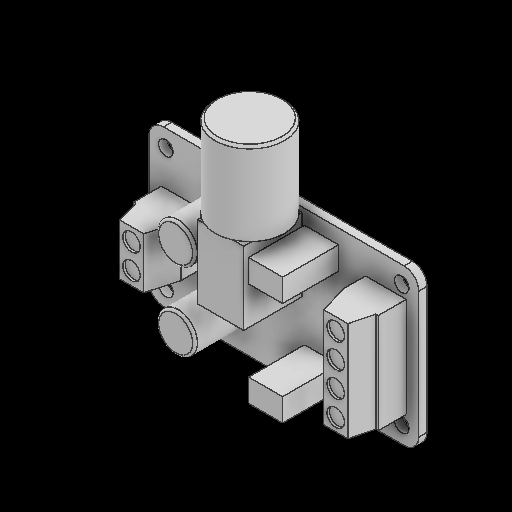
# Autodesk Inventor part: LQ-AMP10W
Saved by Autodesk Inventor 2025.2 (Build 292293000, 293)
## iProperties
Created: 2026-01-28
Part Number: LQ-AMP10W
Material: Generic
Document SubType Name: Modeling
Designer: valer
Density: 1 g/cm^3
Appearance: Default
Author: valer
Autodesk Inventor part; units mm, degrees
ref_plane "YZ Plane" through (0, 0, 0) normal (1, 0, 0) x (0, 1, 0)
ref_plane "XZ Plane" through (0, 0, 0) normal (0, 1, 0) x (-1, 0, 0)
ref_plane "XY Plane" through (0, 0, 0) normal (0, 0, 1) x (1, 0, 0)
sketch "Board" plane through (0, 0, 0) normal (0, 0, 1) x (1, 0, 0)
  line L0 (-27.75, 16) -> (27.75, 16)
  line L1 (27.75, 16) -> (27.75, -16)
  line L2 (27.75, -16) -> (-27.75, -16)
  line L3 (-27.75, -16) -> (-27.75, 16)
  line L4 (-27.75, 16) -> (27.75, -16) construction
  line L5 (27.75, 16) -> (-27.75, -16) construction
  line L6 (-24.25, -12.5) -> (24.25, -12.5) construction
  line L7 (24.25, -12.5) -> (24.25, 12.5) construction
  line L8 (24.25, 12.5) -> (-24.25, 12.5) construction
  line L9 (-24.25, 12.5) -> (-24.25, -12.5) construction
  line L10 (-24.25, -12.5) -> (24.25, 12.5) construction
  line L11 (24.25, -12.5) -> (-24.25, 12.5) construction
  circle A0 centre (24.25, 12.5) radius 1.5
  circle A1 centre (-24.25, 12.5) radius 1.5
  circle A2 centre (24.25, -12.5) radius 1.5
  circle A3 centre (-24.25, -12.5) radius 1.5
  line L12 (-25.75, -14) -> (-22.75, -14) construction
  line L13 (-22.75, -14) -> (-22.75, -11) construction
  line L14 (-22.75, -11) -> (-25.75, -11) construction
  line L15 (-25.75, -11) -> (-25.75, -14) construction
  line L16 (-25.75, -14) -> (-22.75, -11) construction
  line L17 (-22.75, -14) -> (-25.75, -11) construction
  point P0 (0, 0)
  dimension "d0" = 55.5
  dimension "d1" = 32
  dimension "d2" = 3
  dimension "d3" = 2
  dimension "d5" = 2
  dimension "d6" = 48.5
  constraints: 36 end point, 6 midpoint, 6 parallel, 4 centre point, 4 coincident, 3 equal radius, 3 horizontal, 3 perpendicular, 2 tangent
  measures "d0" distance of L0.start L0.end
  measures "d1" distance of L0.end L1.end
  measures "d2" diameter of A0
  measures "d3" distance between parallel lines of L2 L12
  measures "d5" distance between parallel lines of L3 L15
  measures "d6" distance of L7.end L8.end
extrude "BoardFeature" add sketch "Board" along normal blind 1.7
fillet "BoardFilletsFeature" radius 3 4 edges at (-27.75, 16, 0.85) (27.75, 16, 0.85) (-27.75, -16, 0.85) (27.75, -16, 0.85)
sketch "PotentiometerHousing" plane through (0, 0, 1.7) normal (0, 0, 1) x (1, 0, 0)
  line L0 (-5.75, 15) -> (3.75, 15)
  line L1 (3.75, 15) -> (3.75, 0)
  line L2 (3.75, 0) -> (-5.75, 0)
  line L3 (-5.75, 0) -> (-5.75, 15)
  line L4 (24.75, 16) -> (-24.75, 16) projected
  line L5 (-27.75, 13) -> (-27.75, -13) projected
  point P0 (0, 0)
  dimension "d10" = 1
  dimension "d11" = 22
  dimension "d12" = 15
  dimension "d13" = 9.5
  constraints: 8 end point, 2 parallel, 1 horizontal, 1 perpendicular
  measures "d10" distance between parallel lines of L4 L0
  measures "d11" distance between parallel lines of L5 L3
  measures "d12" distance of L0.end L1.end
  measures "d13" distance of L1.end L2.end
extrude "PotentiometerHousingFeature" add sketch "PotentiometerHousing" along normal blind 12
sketch "IJ63" plane through (0, 0, 1.7) normal (0, 0, 1) x (1, 0, 0)
  line L0 (4.25, 13) -> (11.25, 13)
  line L1 (11.25, 13) -> (11.25, 8.3)
  line L2 (11.25, 8.3) -> (4.25, 8.3)
  line L3 (4.25, 8.3) -> (4.25, 13)
  line L4 (3.75, 15) -> (-5.75, 15) projected
  line L5 (3.75, 0) -> (3.75, 15) projected
  line L6 (-38.85, 0) -> (38.85, 0) construction
  line L7 (4.25, -13) -> (11.25, -13)
  line L8 (11.25, -13) -> (11.25, -8.3)
  line L9 (11.25, -8.3) -> (4.25, -8.3)
  line L10 (4.25, -8.3) -> (4.25, -13)
  point P0 (0, 0)
  dimension "d16" = 2
  dimension "d17" = 4.7
  dimension "d18" = 7
  dimension "d19" = 0.5
  constraints: 16 end point, 4 symmetric about line, 2 parallel, 1 horizontal, 1 perpendicular
  measures "d16" distance between parallel lines of L0 L4
  measures "d17" distance between parallel lines of L2 L0
  measures "d18" distance of L1.end L2.end
  measures "d19" distance between parallel lines of L5 L3
extrude "IJ63Feature" add sketch "IJ63" along normal blind 11.5
sketch "Capacitors" plane through (0, 0, 1.7) normal (0, 0, 1) x (1, 0, 0)
  line L0 (-38.85, 0) -> (38.85, 0) construction
  circle A0 centre (-10.75, 8) radius 4
  line L1 (0, -22.4) -> (0, 22.4) construction
  line L2 (-5.75, 15) -> (-5.75, 0) projected
  line L3 (24.75, 16) -> (-24.75, 16) projected
  circle A1 centre (-10.75, -8) radius 4
  point P0 (0, 0)
  dimension "d22" = 8
  dimension "d23" = 5
  dimension "d24" = 8
  constraints: 2 centre point, 1 symmetric about line, 1 other
  measures "d22" diameter of A0
  measures "d23" distance from line of L2 A0.centre
  measures "d24" distance from line of L3 A0.centre
extrude "CapacitorsFeature" add sketch "Capacitors" along normal blind 11.5
sketch "TerminalBlocks" plane through (0, 0, 1.7) normal (0, 0, 1) x (1, 0, 0)
  line L0 (-38.85, 0) -> (38.85, 0) construction
  line L1 (25.18, 10.25) -> (16.83, 10.25)
  line L2 (16.83, 10.25) -> (16.83, -10.25)
  line L3 (16.83, -10.25) -> (25.18, -10.25)
  line L4 (25.18, -10.25) -> (25.18, 10.25)
  line L5 (-25.18, 5.25) -> (-16.83, 5.25)
  line L6 (-16.83, 5.25) -> (-16.83, -5.25)
  line L7 (-16.83, -5.25) -> (-25.18, -5.25)
  line L8 (-25.18, -5.25) -> (-25.18, 5.25)
  line L9 (27.75, -13) -> (27.75, 13) projected
  line L10 (-27.75, 13) -> (-27.75, -13) projected
  point P0 (0, 0)
  point P1 (25.18, 0)
  point P2 (-16.83, 0)
  dimension "d27" = 8.35
  dimension "d28" = 20.5
  dimension "d29" = 10.5
  dimension "d30" = 2.57
  dimension "d31" = 2.57
  constraints: 16 end point, 5 parallel, 2 horizontal, 2 midpoint, 2 perpendicular, 2 point on line
  measures "d27" distance of L1.start L1.end
  measures "d28" distance of L3.end L1.start
  measures "d29" distance of L7.end L5.start
  measures "d30" distance between parallel lines of L9 L4
  measures "d31" distance between parallel lines of L8 L10
extrude "TerminalBlocksFeature" add sketch "TerminalBlocks" along normal blind 10.33
sketch "TerminalBlockProfiles" plane through (16.83, -10.25, 1.7) normal (0, -1, 0) x (1, 0, 0)
  line L0 (8.35, 0) -> (0, 0) projected
  line L1 (8.35, 0) -> (8.35, 10.33) projected
  line L2 (0, 10.33) -> (8.35, 10.33) projected
  line L3 (0, 0) -> (0, 10.33) projected
  line L4 (-33.66, 0) -> (-42.01, 0) projected
  line L5 (-33.66, 0) -> (-33.66, 10.33) projected
  line L6 (-42.01, 10.33) -> (-33.66, 10.33) projected
  line L7 (-42.01, 0) -> (-42.01, 10.33) projected
  line L8 (0, 10.33) -> (8.35, 10.33) projected
  line L9 (1.675, 10.33) -> (0, 4.33)
  line L10 (6.675, 10.33) -> (7.85, 5.72)
  line L11 (7.85, 5.72) -> (8.35, 5.72)
  line L12 (8.35, 0) -> (8.35, 10.33) projected
  line L13 (-16.83, -4.44) -> (-16.83, 14.74) construction
  line L14 (-35.335, 10.33) -> (-33.66, 4.33)
  line L15 (-40.335, 10.33) -> (-41.51, 5.72)
  line L16 (-41.51, 5.72) -> (-42.01, 5.72)
  line L17 (1.675, 10.33) -> (6.675, 10.33)
  point P0 (-16.83, -1.7)
  point P1 (4.175, 10.33)
  point P2 (6.675, 10.33)
  point P3 (1.675, 10.33)
  point P4 (-33.66, 4.33)
  dimension "d34" = 5
  dimension "d35" = 0.5
  dimension "d36" = 4.33
  dimension "d37" = 5.72
  constraints: 14 end point, 5 symmetric about line, 4 point on line, 2 midpoint, 1 collinear, 1 perpendicular
  measures "d34" distance of L10.start L9.start
  measures "d35" distance of L11.end L10.end
  measures "d36" distance from line of L0 L9.end
  measures "d37" distance from line of L0 L11.end
extrude "TerminalBlockProfilesFeature" cut sketch "TerminalBlockProfiles" against normal through all contours L11 L10 L2 L1 | L3 L2 L9 | L14 L6 L5 | L7 L6 L15 L16
sketch "TerminalBlockScrews" plane through (0, 0, 12.03) normal (0, 0, 1) x (1, 0, 0)
  line L0 (18.505, 10.25) -> (18.505, -10.25) projected
  line L1 (18.505, -10.25) -> (23.505, -10.25) projected
  line L2 (23.505, -10.25) -> (23.505, 10.25) projected
  line L3 (23.505, 10.25) -> (18.505, 10.25) projected
  line L4 (-18.505, -5.25) -> (-18.505, 5.25) projected
  line L5 (-18.505, 5.25) -> (-23.505, 5.25) projected
  line L6 (-23.505, 5.25) -> (-23.505, -5.25) projected
  line L7 (-23.505, -5.25) -> (-18.505, -5.25) projected
  line L8 (18.505, 0) -> (23.505, 0) construction
  line L9 (18.505, 0) -> (23.505, 10.25) construction
  line L10 (21.005, 5.125) -> (23.505, 5.125) construction
  line L11 (23.505, 5.125) -> (18.505, 10.25) construction
  circle A0 centre (21.005, 7.6875) radius 1.8
  circle A1 centre (21.005, 2.5625) radius 1.8
  circle A2 centre (21.005, -7.6875) radius 1.8
  line L12 (21.005, 7.6875) -> (21.005, -7.6875) construction
  circle A3 centre (21.005, -2.5625) radius 1.8
  line L13 (0, -22.4) -> (0, 22.4) construction
  circle A4 centre (-21.005, 2.5625) radius 1.8
  circle A5 centre (-21.005, -2.5625) radius 1.8
  point P0 (0, 0)
  dimension "d41" = 3.6
  dimension "d42" = 2.5625
  dimension "d43" = 2.5625
  constraints: 10 end point, 6 centre point, 4 midpoint, 4 symmetric about line, 2 point on line, 1 equal radius, 1 parallel, 1 perpendicular, 4 other
  measures "d41" diameter of A0
  measures "d42" distance from line of L3 L12.start
  measures "d43" distance from line of L8 A1.centre
extrude "TerminalBlockScrewsFeature" cut sketch "TerminalBlockScrews" against normal blind 0.5 contours A0 | A1 | A2 | A3 | A4 | A5
fillet "FilletsFeature" radius 0.5 2 edges at (-14.75, -8, 13.2) (-14.75, 8, 13.2)
sketch "PotentiometerShaft" plane through (-5.75, 15, 1.7) normal (0, 1, 0) x (1, 0, 0)
  line L0 (0, 0) -> (9.5, 0) projected
  line L1 (0, 0) -> (0, -12) projected
  line L2 (9.5, -12) -> (0, -12) projected
  line L3 (9.5, 0) -> (9.5, -12) projected
  line L4 (9.5, -12) -> (0, 0) construction
  circle A0 centre (4.75, -6) radius 3
  point P0 (5.75, 1.7)
  dimension "d48" = 6
  constraints: 2 end point, 1 centre point, 1 midpoint
  measures "d48" diameter of A0
extrude "PotentiometerShaftFeature" add sketch "PotentiometerShaft" along normal blind 0.5 contours A0
sketch "PotentiometerKnob" plane through (-1, 15.5, 7.7) normal (0, 1, 0) x (1, 0, 0)
  circle A0 centre (0, 0) radius 3 projected
  circle A1 centre (0, 0) radius 3 projected
  circle A2 centre (0, 0) radius 7.15
  point P0 (1, 7.7)
  dimension "d51" = 14.3
  constraints: 1 centre point, 1 coincident
  measures "d51" diameter of A2
extrude "PotentiometerKnobFeature" add sketch "PotentiometerKnob" along normal blind 17 contours A0 | A2
chamfer "PotentiometerKnobChamferFeature" distance 0.5 angle 45 1 edges at (-8.15, 32.5, 7.7)
equation "\"d5\" = d3"
equation "\"d31\" = d30"
equation "\"d43\" = d42"
body "Solid1"
